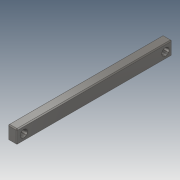
# Autodesk Inventor part: 200-60-DIFFERENTIAL-BAR-05
Saved by Autodesk Inventor 2018.2 (Build 222227000, 227)
## iProperties
Manager: feesmrt
Company: FRANCOR
Part Number: 200-60-DIFFERENTIAL-BAR-05
Project: Rescue Robot
Cost Center: -
Material: Edelstahl
Document SubType Name: Modeling
Designer: feesmrt
Engineer: feesmrt
Authority: feesmrt
Density: 8 g/cm^3
Appearance: Halbpoliert
Description: Differential Verbindungsstange
Stock Number: 200-60-DIFFERENTIAL-BAR-05
Subject: Rescue Robot
Author: feesmrt
Revision Number: 1
Title: Differential Verbindungsstange
Autodesk Inventor part; units mm, degrees
ref_plane "YZ Plane" through (0, 0, 0) normal (1, 0, 0) x (0, 1, 0)
ref_plane "XZ Plane" through (0, 0, 0) normal (0, 1, 0) x (-1, 0, 0)
ref_plane "XY Plane" through (0, 0, 0) normal (0, 0, 1) x (1, 0, 0)
sketch "Skizze1" plane through (0, 0, 0) normal (0, 0, 1) x (1, 0, 0)
  line L0 (-5, -85) -> (5, -85)
  line L1 (5, -85) -> (5, 85)
  line L2 (5, 85) -> (-5, 85)
  line L3 (-5, 85) -> (-5, -85)
  line L4 (-5, -85) -> (5, 85) construction
  line L5 (5, -85) -> (-5, 85) construction
  point P0 (0, 0)
  dimension "d0" = 10
  dimension "d1" = 170
  constraints: 12 end point, 2 midpoint, 2 parallel, 1 horizontal, 1 perpendicular
  measures "d0" distance between parallel lines of L1 L3
  measures "d1" distance between parallel lines of L0 L2
extrude "Grundkörper" add sketch "Skizze1" along normal mid plane 15
sketch "Skizze2" plane through (5, -85, 7.5) normal (1, 0, 0) x (0, 0, -1)
  line L0 (7.5, -34) -> (7.5, 204) projected
  line L1 (-3, 85) -> (18, 85) projected
  point P0 (7.5, 85)
  point P1 (7.5, 7.5)
  point P2 (7.5, 162.5)
  dimension "d4" = 155
  constraints: 2 point on line, 1 symmetric about line
  measures "d4" distance of point (7.5, 162.5) point (7.5, 7.5)
hole "Boh_8" at (5, -77.5, 0) at (5, 77.5, 0) direction (-1, 0, 0) diameter 8.1 end through all
chamfer "Fase_Allgemein" distance 1 angle 45 12 edges at (5, 0, 7.5) (-5, 0, 7.5) (5, 0, -7.5) (-5, 0, -7.5) (0, -85, 7.5) (0, -85, -7.5) (5, -85, 0) (-5, -85, 0) (0, 85, 7.5) (5, 85, 0) (0, 85, -7.5) (-5, 85, 0)
